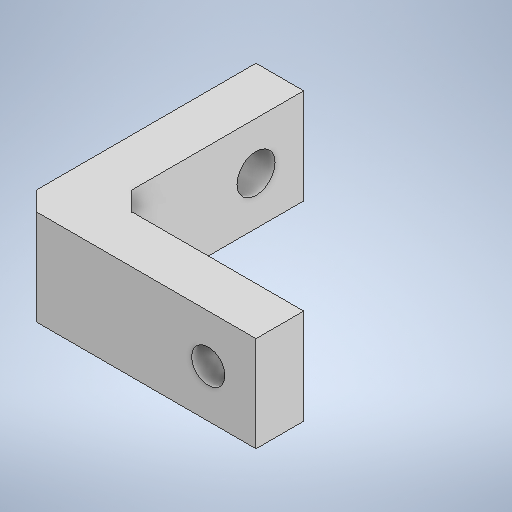
# Autodesk Inventor part: L connection
Saved by Autodesk Inventor 2025.3 (Build 293356000, 356)
## iProperties
Created: 2025-12-09
Part Number: L connection
Material: Generic
Document SubType Name: Modeling
Designer: hazem
Density: 1 g/cm^3
Appearance: Default
Author: hazem
Autodesk Inventor part; units mm, degrees
ref_plane "YZ Plane" through (0, 0, 0) normal (1, 0, 0) x (0, 1, 0)
ref_plane "XZ Plane" through (0, 0, 0) normal (0, 1, 0) x (-1, 0, 0)
ref_plane "XY Plane" through (0, 0, 0) normal (0, 0, 1) x (1, 0, 0)
sketch "Sketch1" plane through (0, 0, 0) normal (0, 1, 0) x (-1, 0, 0)
  line L0 (0, 0) -> (25, 0)
  line L1 (25, 0) -> (25, -25)
  line L2 (25, -25) -> (20, -25)
  line L3 (20, -25) -> (20, -5)
  line L4 (20, -5) -> (0, -5)
  line L5 (0, -5) -> (0, 0)
  dimension "d0" = 5
  dimension "d1" = 25
  dimension "d2" = 25
  constraints: 12 end point, 6 perpendicular, 1 horizontal
  measures "d0" distance of L4.end L0.start
  measures "d1" distance of L0.start L0.end
  measures "d2" distance of L0.end L1.end
extrude "Extrusion1" add sketch "Sketch1" along normal mid plane 10
sketch "Sketch2" plane through (-20, -5, -25) normal (1, 0, 0) x (0, 0, -1)
  circle A0 centre (-5, 5) radius 2
  line L0 (-25, 0) -> (-25, 10) projected
  line L1 (-20, 10) -> (0, 10) projected
  line L2 (0, 0) -> (0, 10) projected
  point P0 (-25, 5)
  point P1 (-25, 5)
  dimension "d5" = 4
  dimension "d9" = 5
  constraints: 1 centre point, 1 horizontal alignment, 1 midpoint
  measures "d5" diameter of A0
  measures "d9" distance from line of L2 A0.centre
extrude "Extrusion2" cut sketch "Sketch2" against normal through all
sketch "Sketch3" plane through (0, 5, -5) normal (0, 0, -1) x (-1, 0, 0)
  circle A0 centre (5, -5) radius 1.75
  line L0 (0, 0) -> (0, -10) projected
  line L1 (0, 0) -> (20, 0) projected
  point P0 (0, -5)
  point P1 (0, -5)
  point P2 (0, -5)
  dimension "d8" = 3.5
  dimension "d11" = 5
  constraints: 2 midpoint, 1 centre point, 1 horizontal alignment
  measures "d8" diameter of A0
  measures "d11" distance from line of L0 A0.centre
extrude "Extrusion3" cut sketch "Sketch3" against normal blind 10
chamfer "Chamfer1" distance 2 angle 45 2 edges at (-25, 0, 0) (-20, 0, -5)
body "Solid1"
